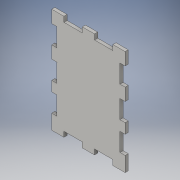
# Autodesk Inventor part: bottom
Saved by Autodesk Inventor 2016 (Build 200138000, 138)
## iProperties
Created: 2016-05-17
Part Number: bottom
Material: Generic
Document SubType Name: Modeling
Designer: Lillahunden
Density: 1 g/cm^3
Appearance: Default
Author: Lillahunden
Autodesk Inventor part; units mm, degrees
ref_plane "YZ Plane" through (0, 0, 0) normal (1, 0, 0) x (0, 1, 0)
ref_plane "XZ Plane" through (0, 0, 0) normal (0, 1, 0) x (-1, 0, 0)
ref_plane "XY Plane" through (0, 0, 0) normal (0, 0, 1) x (1, 0, 0)
sketch "Sketch1" plane through (0, 0, 0) normal (0, 1, 0) x (-1, 0, 0)
  line L0 (-70, 100) -> (70, -100) construction
  line L1 (70, 100) -> (-70, -100) construction
  line L2 (70, 17.5) -> (60, 17.5)
  line L3 (60, 17.5) -> (60, -17.5)
  line L4 (60, -17.5) -> (70, -17.5)
  line L5 (70, -17.5) -> (70, 17.5) construction
  line L6 (70, 76.25) -> (60.2105, 76.25)
  line L7 (60.2105, 76.25) -> (60.2105, 41.25)
  line L8 (60.2105, 41.25) -> (70, 41.25)
  line L9 (70, -36.6283) -> (60.2105, -36.6283)
  line L10 (60.2105, -36.6283) -> (60.2105, -71.6283)
  line L11 (60.2105, -71.6283) -> (70, -71.6283)
  line L12 (70, 100) -> (70, 76.25)
  line L13 (70, 41.25) -> (70, -36.6283) construction
  line L14 (70, -71.6283) -> (70, -100)
  line L15 (70, 17.5) -> (70, 41.25)
  line L16 (70, -17.5) -> (70, -36.6283)
  line L17 (11.66, -100) -> (10.1921, -100)
  line L18 (-46.67, -100) -> (-48.1379, -100)
  line L19 (70, -100) -> (46.67, -100)
  line L20 (10.1921, -100) -> (-70, -100) construction
  line L21 (46.67, -102.534) -> (46.67, -125.8746) construction
  line L22 (11.66, -102.534) -> (11.66, -137.131) construction
  line L23 (-11.67, -101.9546) -> (-11.67, -114.6181) construction
  line L24 (-46.67, -61.1499) -> (-46.67, -142.7592) construction
  line L25 (11.66, -100) -> (11.66, -90)
  line L26 (11.66, -90) -> (46.67, -90)
  line L27 (46.67, -90) -> (46.67, -100)
  line L28 (-11.67, -100) -> (-46.67, -100) construction
  line L29 (-46.67, -100) -> (-46.67, -90) construction
  line L30 (-46.67, -90) -> (-11.67, -90)
  line L31 (-11.67, -90) -> (-11.67, -100)
  line L32 (-46.67, -90) -> (-46.67, -100)
  line L33 (-70, -100) -> (-46.67, -100)
  line L34 (11.66, -100) -> (-11.67, -100)
  line L35 (0, 0) -> (69.1947, 0) construction
  line L36 (-70, -100) -> (70, 100) construction
  line L37 (70, -100) -> (-70, 100) construction
  line L38 (11.66, 100) -> (10.1921, 100)
  line L39 (-46.67, 100) -> (-48.1379, 100)
  line L40 (70, 100) -> (46.67, 100)
  line L41 (10.1921, 100) -> (-70, 100) construction
  line L42 (46.67, 102.534) -> (46.67, 125.8746) construction
  line L43 (11.66, 102.534) -> (11.66, 137.131) construction
  line L44 (-11.67, 101.9546) -> (-11.67, 114.6181) construction
  line L45 (-46.67, 61.1499) -> (-46.67, 142.7592) construction
  line L46 (11.66, 100) -> (11.66, 90)
  line L47 (11.66, 90) -> (46.67, 90)
  line L48 (46.67, 90) -> (46.67, 100)
  line L49 (-46.67, 100) -> (-46.67, 90) construction
  line L50 (-46.67, 90) -> (-11.67, 90)
  line L51 (-11.67, 90) -> (-11.67, 100)
  line L52 (-46.67, 90) -> (-46.67, 100)
  line L53 (-70, 100) -> (-46.67, 100)
  line L54 (11.66, 100) -> (-11.67, 100)
  line L55 (-0.0025, -36.6283) -> (-0.0025, 49.5513) construction
  line L56 (69.995, 100) -> (-70.005, -100) construction
  line L57 (-70.005, 100) -> (69.995, -100) construction
  line L58 (-70.005, 17.5) -> (-60.005, 17.5)
  line L59 (-60.005, 17.5) -> (-60.005, -17.5)
  line L60 (-60.005, -17.5) -> (-70.005, -17.5)
  line L61 (-70.005, 0) -> (-70.005, 17.5) construction
  line L62 (-70.005, 76.25) -> (-60.2155, 76.25)
  line L63 (-60.2155, 76.25) -> (-60.2155, 41.25)
  line L64 (-60.2155, 41.25) -> (-70.005, 41.25)
  line L65 (-70.005, -36.6283) -> (-60.2155, -36.6283)
  line L66 (-60.2155, -36.6283) -> (-60.2155, -71.6283)
  line L67 (-60.2155, -71.6283) -> (-70.005, -71.6283)
  line L68 (-70.005, 100) -> (-70.005, 76.25)
  line L69 (-70.005, -71.6283) -> (-70.005, -100)
  line L70 (-70.005, 17.5) -> (-70.005, 41.25)
  line L71 (-70.005, -17.5) -> (-70.005, -36.6283)
  line L72 (-0.005, 0) -> (-69.1997, 0) construction
  line L73 (-70.005, -100) -> (69.995, 100) construction
  line L74 (69.995, -100) -> (-70.005, 100) construction
  line L75 (-70, 76.25) -> (-70, 100)
  line L76 (-70.005, 41.25) -> (-70.005, 17.5) construction
  line L77 (-70.005, -17.5) -> (-70.005, -36.6283) construction
  line L78 (-70, 17.5) -> (-70, 41.25)
  line L79 (-70, -100) -> (-70, -71.6283)
  line L80 (-70, -36.6283) -> (-70, -17.5)
  line L81 (-70, 100) -> (-46.67, 100)
  line L82 (-11.67, 100) -> (11.66, 100)
  line L83 (46.67, 100) -> (70, 100)
  point P0 (70, 0)
  point P1 (0, 0)
  point P2 (-30.6379, -100)
  point P3 (-46.67, -101.9546)
  point P4 (-30.6379, 100)
  point P5 (-46.67, 101.9546)
  dimension "d0" = 140
  dimension "d2" = 10
  dimension "d3" = 35
  dimension "d4" = 35
  dimension "d5" = 35
  dimension "d8" = 23.75
  dimension "d9" = 19.1283
  dimension "d17" = 23.33
  dimension "d18" = 23.33
  dimension "d19" = 35
  dimension "d20" = 35.01
  dimension "d21" = 10
  dimension "d22" = 10
  dimension "d27" = 200
  constraints: 168 end point, 47 symmetric about line, 25 parallel, 20 point on line, 13 perpendicular, 9 horizontal, 7 midpoint, 5 vertical, 4 horizontal alignment, 3 collinear
  measures "d0" distance of L0.end L1.end
  measures "d2" distance of L4.end L3.end
  measures "d3" distance of L3.end L2.end
  measures "d4" distance of L7.end L6.end
  measures "d5" distance of L10.end L9.end
  measures "d8" distance between parallel lines of L8 L2
  measures "d9" distance between parallel lines of L9 L4
  measures "d17" distance between parallel lines of L23 L22
  measures "d18" distance between parallel lines of L21 L14
  measures "d19" distance between parallel lines of L23 L24
  measures "d20" distance between parallel lines of L21 L22
  measures "d21" distance of L17.start L25.end
  measures "d22" distance of L18.start L29.end
  measures "d27" distance between parallel lines of L53 L20
extrude "Extrusion1" add sketch "Sketch1" along normal blind 6 contours L2 L3 L4 L16 L9 L10 L11 L14 L19 L27 L26 L25 L17 L34 L31 L30 L32 L18 L33 L79 L67 L66 L65 L80 L60 L59 L58 L78 L64 L63 L62 L75 L53 L39 L52 L50 L51 L54 L38 L46 L47 L48 L40 L12 L6 L7 L8 L15
equation "\"d7\" = d6"
equation "\"d6\" = 23.75"
body "Solid1"
